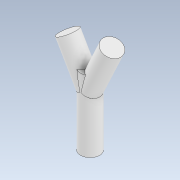
# Autodesk Inventor part: 珊瑚
Saved by Autodesk Inventor 2022.5 (Build 265521000, 521)
## iProperties
Created: 2024-11-12
Part Number: 珊瑚
Material: 聚苯乙烯
Document SubType Name: Modeling
Designer: Gagouking
Mass: 113.944 g
Surface Area: 176.848 cm^2
Volume: 111.601 cm^3
Density: 1.021 g/cm^3
Appearance: 平滑 - 白色
Author: Gagouking
Autodesk Inventor part; units mm, degrees
ref_plane "YZ Plane" through (0, 0, 0) normal (1, 0, 0) x (0, 1, 0)
ref_plane "XZ Plane" through (0, 0, 0) normal (0, 1, 0) x (-1, 0, 0)
ref_plane "XY Plane" through (0, 0, 0) normal (0, 0, 1) x (1, 0, 0)
sketch "草图1" plane through (0, 0, 0) normal (0, 1, 0) x (-1, 0, 0)
  circle A0 centre (0, 0) radius 13.45
  dimension "d0" = 26.9
  constraints: 1 centre point, 1 coincident
  measures "d0" diameter of A0
extrude "拉伸1" add sketch "草图1" along normal blind 100
sketch "草图2" plane through (0, 100, 0) normal (0, 1, 0) x (1, 0, 0)
  line L0 (40, -45.1945) -> (40, 45.1945)
  line L1 (0, 0) -> (40, 0) construction
  line L2 (-50, 47.95) -> (-50, -45.1945)
  dimension "d3" = 40
  dimension "d7" = 50
  constraints: 6 end point, 2 vertical, 1 horizontal, 1 midpoint
  measures "d3" distance of L1.end L1.start
  measures "d7" distance from line of L2 L1.start
ref_plane "工作平面1" through (40, 100, 45.1945) normal (0.5, -0.8660254, 0) x (0, 0, -1)
sketch "草图3" plane through (40, 100, 45.1945) normal (0.5, -0.8660254, 0) x (0, 0, -1)
  circle A0 centre (45.1945, -47.9023) radius 13.45
  line L0 (31.7445, -84.641) -> (31.7445, -34.641) projected
  line L1 (58.6445, -84.641) -> (58.6445, -34.641) projected
  point P0 (45.1945, -84.641)
  constraints: 2 tangent, 1 centre point
extrude "拉伸2" add sketch "草图3" against normal blind 60
ref_plane "工作平面2" through (-50, 100, -47.95) normal (-0.4226183, -0.9063078, 0) x (0, 0, 1)
sketch "草图4" plane through (-50, 100, -47.95) normal (-0.4226183, -0.9063078, 0) x (0, 0, 1)
  circle A0 centre (47.95, -56.336) radius 13.45
  line L0 (61.4, -87.5772) -> (61.4, -45.3154) projected
  line L1 (34.5, -87.5772) -> (34.5, -45.3154) projected
  point P0 (47.95, -87.5772)
  constraints: 2 tangent, 1 centre point
extrude "拉伸3" add sketch "草图4" against normal blind 70
